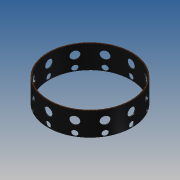
# Autodesk Inventor part: 2h1sout
Saved by Autodesk Inventor 2014 SP1 (Build 180222100, 222)
## iProperties
Company: HERA Project
Created: 2013-05-14
Part Number: 2h1sout
Material: Generic
Document SubType Name: Modeling
Designer: David DeBoer
Density: 1 g/cm^3
Description: Hub outer sonotube
Appearance: Default
Author: David DeBoer
Title: Hub outer sono
Autodesk Inventor part; units mm, degrees
ref_plane "YZ Plane" through (0, 0, 0) normal (1, 0, 0) x (0, 1, 0)
ref_plane "XZ Plane" through (0, 0, 0) normal (0, 1, 0) x (-1, 0, 0)
ref_plane "XY Plane" through (0, 0, 0) normal (0, 0, 1) x (1, 0, 0)
sketch "Sketch1" plane through (0, 0, 0) normal (0, 1, 0) x (-1, 0, 0)
  circle A0 centre (0, 0) radius 457.2
  circle A1 centre (0, 0) radius 444.5
  dimension "d0" = 914.4
  dimension "d2" = 12.7
  constraints: 2 centre point, 1 coincident
  measures "d0" diameter of A0
  measures "d2" radial gap between concentric circles of A1 A0
extrude "tube" add sketch "Sketch1" along normal blind 254
sketch "Sketch2" plane through (0, 0, 0) normal (0, -1, 0) x (1, 0, 0)
  circle A0 centre (0, 0) radius 444.5 projected
  circle A1 centre (0, 0) radius 457.2 projected
  point P0 (-457.2, 0)
  constraints: 1 horizontal alignment, 1 other
ref_plane "Work Plane1" through (-457.2, 0, 0) normal (-1, 0, 0) x (0, -1, 0)
sketch "Sketch3" plane through (-457.2, 0, 0) normal (-1, 0, 0) x (0, -1, 0)
  circle A0 centre (-149.86, 0) radius 12.7
  line L0 (0, -457.2) -> (0, 457.2) projected
  line L1 (-254, 457.2) -> (-254, -457.2) projected
  point P0 (0, 0)
  dimension "d5" = 25.4
  dimension "d7" = 149.86
  dimension "d67" = 104.14
  constraints: 1 centre point
  measures "d5" diameter of A0
  measures "d7" distance from line of A0.centre L0
  measures "d67" distance from line of A0.centre L1
hole "spar" at (-457.2, 149.86, 0) direction (1, 0, 0) diameter 88.9 end through all
pattern_circular "spar pattern" count 12 over 360 about axis through (0, 0, 0) along (0, 1, 0) of "spar"
sketch "Sketch4" plane through (0, 254, 0) normal (0, 1, 0) x (1, 0, 0)
  circle A0 centre (0, 0) radius 444.5 projected
  circle A1 centre (0, 0) radius 457.2 projected
  line L0 (-6.8782, 0) -> (527.6153, -106.3174) construction
  line L1 (-6.8782, 0) -> (538.0866, 0) construction
  point P0 (448.1513, -90.511)
  dimension "d18" = 11.25
  constraints: 4 end point, 1 equal length, 1 horizontal, 1 point on line, 2 other
  measures "d18" angle of L0 L1
ref_plane "Work Plane2" through (448.1513, 254, 90.511) normal (0.9807853, 0, 0.1950903) x (0, 1, 0)
sketch "Sketch7" plane through (-457.2, 0, 0) normal (-1, 0, 0) x (0, -1, 0)
  circle A0 centre (-30.48, 0) radius 30.1625
  point P0 (0, 0)
  dimension "d32" = 60.325
  dimension "d33" = 30.48
  constraints: 1 centre point
  measures "d32" diameter of A0
  measures "d33" distance of point (0, 0) A0.centre
hole "support" at (-457.2, 30.48, 0) direction (1, 0, 0) diameter 60.325 end through all
pattern_circular "support pattern" count 12 over 360 about axis through (0, 0, 0) along (0, 1, 0) of "support"
sketch "Sketch8" plane through (0, 254, 0) normal (0, 1, 0) x (1, 0, 0)
  circle A0 centre (0, 0) radius 444.5 projected
  circle A1 centre (0, 0) radius 457.2 projected
  point P0 (320.675, -325.8825)
  constraints: 2 other
sketch "Sketch10" plane through (0, 254, 0) normal (0, 1, 0) x (1, 0, 0)
  circle A0 centre (0, 0) radius 444.5 projected
  circle A1 centre (0, 0) radius 457.2 projected
  point P0 (0, -457.2)
  constraints: 1 vertical alignment, 1 other
ref_plane "Work Plane5" through (0, 254, 0) normal (0, 0, 1) x (1, 0, 0)
ref_plane "Work Plane4" through (0, 254, 457.2) normal (0, 0, 1) x (1, 0, 0)
sketch "Sketch13" plane through (0, 0, 0) normal (0, -1, 0) x (1, 0, 0)
  circle A0 centre (0, 0) radius 444.5 projected
  circle A1 centre (0, 0) radius 457.2 projected
  point P0 (0, -457.2)
  constraints: 1 vertical alignment, 1 other
ref_plane "Work Plane6" through (0, 0, -457.2) normal (0, 0, -1) x (-1, 0, 0)
sketch "Sketch14" plane through (0, 0, -457.2) normal (0, 0, -1) x (-1, 0, 0)
  line L0 (-1.27, 0) -> (1.27, 0)
  line L1 (1.27, 0) -> (1.27, 0.762)
  line L2 (1.27, 0.762) -> (-1.27, 0.762)
  line L3 (-1.27, 0.762) -> (-1.27, 0)
  line L4 (0, 0.762) -> (0, 0) construction
  line L5 (0, 0) -> (0, 1.4167) construction
  dimension "d56" = 2.54
  dimension "d57" = 0.762
  constraints: 12 end point, 2 collinear, 2 midpoint, 2 parallel, 1 horizontal, 1 perpendicular
  measures "d56" distance of L2.end L1.end
  measures "d57" distance of L1.end L0.end
extrude "ALIGNMENT_hub" add sketch "Sketch14" along normal blind 0.635
sketch "Sketch15" plane through (0, 254, 0) normal (0, 1, 0) x (1, 0, 0)
  circle A0 centre (0, 0) radius 444.5 projected
  circle A1 centre (0, 0) radius 457.2 projected
  point P0 (0, 457.2)
  constraints: 1 vertical alignment, 1 other
ref_plane "Work Plane7" through (0, 254, -457.2) normal (0, 0, -1) x (-1, 0, 0)
sketch "Sketch16" plane through (0, 254, -457.2) normal (0, 0, -1) x (-1, 0, 0)
  circle A0 centre (0, -223.52) radius 30.1625
  line L0 (-457.2, -254) -> (457.2, -254) projected
  circle A1 centre (0, -223.52) radius 31.4325
  point P0 (0, -254)
  dimension "d60" = 30.48
  dimension "d61" = 60.325
  dimension "d62" = 1.27
  constraints: 2 centre point
  measures "d60" distance from line of L0 A0.centre
  measures "d61" diameter of A0
  measures "d62" radial gap between concentric circles of A1 A0
extrude "ALIGNMENT_SUPPORT" add sketch "Sketch16" against normal blind 12.7
sketch "Sketch17" plane through (0, 254, -457.2) normal (0, 0, -1) x (-1, 0, 0)
  line L0 (0, 0) -> (79.1926, 0) construction
  point P0 (0, -254)
  constraints: 2 end point, 1 horizontal
ref_plane "Work Plane8" through (0, 254, -457.2) normal (0, 0, -1) x (-1, 0, 0)
sketch "Sketch18" plane through (0, 254, -457.2) normal (0, 0, -1) x (-1, 0, 0)
  circle A0 centre (0, -104.14) radius 44.45
  line L0 (-1.27, -254) -> (1.27, -254) projected
  circle A1 centre (0, -104.14) radius 46.99
  point P0 (0, -254)
  point P1 (0, -253.6558)
  point P2 (1.27, -254)
  dimension "d66" = 88.9
  dimension "d70" = 149.86
  dimension "d71" = 2.54
  constraints: 2 centre point, 1 other
  measures "d66" diameter of A0
  measures "d71" radial gap between concentric circles of A1 A0
extrude "ALIGNMENT_SPAR" add sketch "Sketch18" against normal blind 12.7
body "Solid1"
